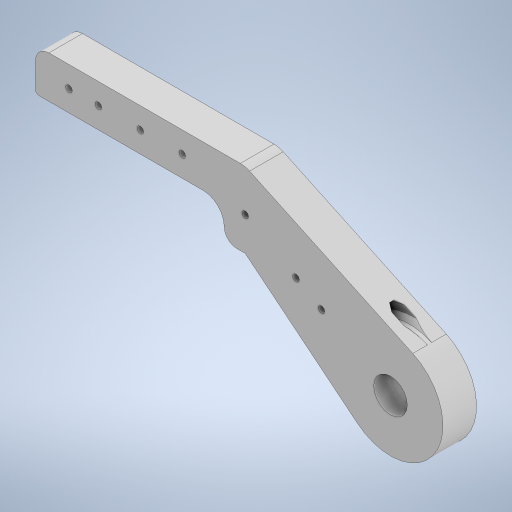
# Autodesk Inventor part: palec1
Saved by Autodesk Inventor 2024.2 (Build 282272000, 272)
## iProperties
Created: 2023-12-27
Part Number: palec1
Material: PLA
Document SubType Name: Modeling
Designer: Konrad
Density: 1 g/cm^3
Appearance: Domyślna
Author: Konrad
Autodesk Inventor part; units mm, degrees
ref_plane "YZ Plane" through (0, 0, 0) normal (1, 0, 0) x (0, 1, 0)
ref_plane "XZ Plane" through (0, 0, 0) normal (0, 1, 0) x (-1, 0, 0)
ref_plane "XY Plane" through (0, 0, 0) normal (0, 0, 1) x (1, 0, 0)
sketch "Szkic1" plane through (0, 0, 0) normal (0, 0, 1) x (1, 0, 0)
  circle A0 centre (0, 0) radius 4
  circle A1 centre (0, 0) radius 12.5
  line L0 (0, 0) -> (-34.641016, 20) construction
  line L1 (-44.641016, 20) -> (-84.641016, 20)
  line L2 (-34.641016, 20) -> (-34.641016, 30) construction
  line L3 (-34.641016, 30) -> (5.295397, 11.322931)
  line L4 (-34.641016, 20) -> (-34.641016, 12) construction
  line L5 (-34.641016, 12) -> (-7.873676, -9.708513)
  line L6 (-84.641016, 20) -> (-84.641016, 30)
  line L7 (-84.641016, 30) -> (-34.641016, 30)
  line L8 (-34.641016, 12) -> (-39.641016, 12)
  line L9 (-39.641016, 12) -> (-39.641016, 15)
  line L10 (-39.641016, 20) -> (-34.641016, 30)
  line L11 (-42.641016, 20) -> (-37.641016, 30)
  arc A2 (-3.751618, 15.55395) -> (-15.630772, -3.41745) centre (0, 0) ccw
  line L12 (-104.069219, 0) -> (31.928203, 0) construction
  line L13 (-20.484833, 0.519229) -> (-10.092448, 18.519367) construction
  line L14 (-39.641016, 12) -> (-44.641016, 12)
  line L15 (-44.641016, 12) -> (-44.641016, 15)
  line L16 (-44.641016, 15) -> (-39.641016, 15)
  arc A3 (-39.641016, 15) -> (-44.641016, 20) centre (-44.641016, 15) ccw
  arc A4 (-39.641016, 15) -> (-36.641016, 12) centre (-36.641016, 15) ccw
  circle A5 centre (-76.641016, 25) radius 0.8
  circle A6 centre (-69.641016, 25) radius 0.8
  line L17 (-76.641016, 25) -> (-69.641016, 25) construction
  circle A7 centre (-59.641016, 25) radius 0.8
  circle A8 centre (-49.641016, 25) radius 0.8
  circle A9 centre (-16.454483, 9.5) radius 0.8
  circle A10 centre (-22.51666, 13) radius 0.8
  circle A11 centre (-34.641016, 20) radius 0.8
  dimension "d0" = 25
  dimension "d1" = 32
  dimension "d2" = 8
  dimension "d4" = 40
  dimension "d5" = 30
  dimension "d6" = 50
  dimension "d7" = 10
  dimension "d8" = 5
  dimension "d9" = 3
  dimension "d10" = 8
  dimension "d11" = 22
  dimension "d16" = 5
  dimension "d17" = 3
  dimension "d20" = 5
  dimension "d21" = 3
  dimension "d23" = 1.6
  dimension "d25" = 8
  dimension "d26" = 5
  dimension "d27" = 15
  dimension "d31" = 10
  dimension "d38" = 19
  dimension "d39" = 7
  constraints: 34 end point, 15 point on line, 12 centre point, 8 point on circle, 5 horizontal, 5 perpendicular, 4 coincident, 4 equal radius, 4 tangent, 2 vertical, 1 parallel, 4 other
  measures "d0" diameter of A1
  measures "d1" diameter of A2
  measures "d2" diameter of A0
  measures "d4" distance of L0.start L0.end
  measures "d5" angle of L12 L0
  measures "d6" distance of L0.end L1.end
  measures "d7" distance of L1.end L6.end
  measures "d8" distance of L4.end L8.end
  measures "d9" distance of L11.end L2.end
  measures "d10" distance of L8.end L10.start
  measures "d11" distance from line of L0.end L13
  measures "d16" distance of L8.end L14.end
  measures "d17" distance of L14.end L15.end
  measures "d20" radius of A3
  measures "d21" radius of A4
  measures "d23" diameter of A5
  measures "d25" distance from line of L6 L17.start
  measures "d26" distance from line of L7 L17.start
  measures "d27" distance from line of L6 L17.end
  measures "d31" distance of L17.end A7.centre
  measures "d38" distance of point (0, 0) A9.centre
  measures "d39" distance of A9.centre A10.centre
extrude "Wyciągnięcie proste1" add sketch "Szkic1" along normal mid plane 8 contours A1 | A1 L5 A2 L3 | A2 L5 L8 A4 A3 L1 L6 L7 L3
extrude "Wyciągnięcie proste2" cut sketch "Szkic1" along normal mid plane 3 contours A1 L5 A2 L3
fillet "Zaokrąglenie2" radius 3.2 1 edges at (-84.641, 30, 0)
fillet "Zaokrąglenie3" radius 5.2 1 edges at (-34.641, 30, 0)
chamfer "Faza1" distance 1 angle 45 4 edges at (-13.5609, 8.4913, -1.5) (-13.5609, 8.4913, 1.5) (-10.5944, 6.6338, -1.5) (-10.5944, 6.6338, 1.5)
fillet "Zaokrąglenie4" radius 0.8 1 edges at (-84.641, 20, 0)
